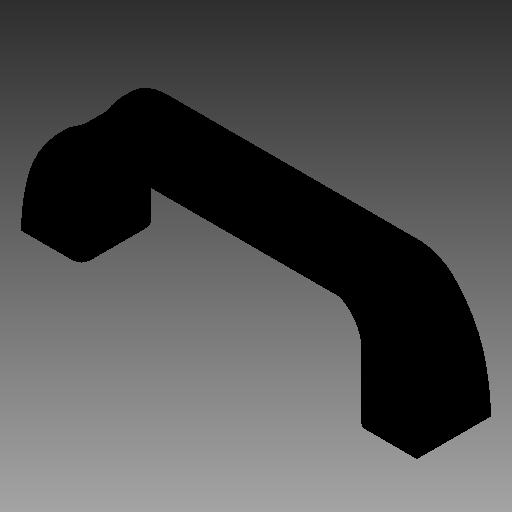
# Autodesk Inventor part: 2061
Saved by Autodesk Inventor 2019 (Build 230136000, 136)
## iProperties
Category: PARTsolutions
Company: 8020
Created: 2019-03-04
Part Number: 2061
Material: Generic
Catalog Web Link: www.cadenas.de
Description: 2060, 2061, 2062, 2880, 2881, 2882-Plastic Door Handles
Vendor: 8020
Document SubType Name: Modeling
Designer: psadmin
Manufacturer: 8020
Mass: 38.2907 g
Surface Area: 160.706 cm^2
Volume: 38.2907 cm^3
Density: 1 g/cm^3
Appearance: PSOLRGB-0-0-0
PSOL_IDENT_0: {$CADENAS_DATA\23d-libs\8020\inch\panels_and_doors\2060.prj},182 {VTYP=3D},{NB=2061},{LINA=2061},{NN=
PSOL_IDENT_1: 2060, 2061, 2062, 2880, 2881, 2882},{DATE=04.12.2018 10:30:17},{GEOMDATE=03.01.2012 00:00:00},{VERSI
PSOL_IDENT_2: ON=},{LINEID=300},{WBVAR=COLOR},{WBNUMERIC=}  {NB=2061},{LINA=2061},{KT=DUMMY},{PN=2061},{SIZE=Mediu
PSOL_IDENT_3: m},{MAT=High Strength Polycarbonate},{COLOR=Black},{A=5.473},{B=3.800},{C=1.614},{D=1.024},{E=4.607}
PSOL_IDENT_4: ,{F=5/16-18 SHCS (2)},{W=.095},{CC=8-15, 8-40},{COL=0.00,0.00,0.00,0.00}
NN: 2060, 2061, 2062, 2880, 2881, 2882
NT: Plastic Door Handles
NB: 2061
NBSYN: $PN.
LINA: 2061
PN: 2061
SIZE: Medium
MAT: High Strength Polycarbonate
COLOR: Black
A: 5.473
B: 3.8
C: 1.614
D: 1.024
E: 4.607
F: 5/16-18 SHCS (2)
W: .095
CC: 8-15, 8-40
SUPPLIER: 8020
ARTICLENO: 2061
BOMINFO: 2061
CREATOR: CADENAS GmbH
Title: 2061
Author: Cadenas PARTsolutions
Comments: Plastic Door Handles
Autodesk Inventor part; units mm, degrees
ref_plane "YZ Plane" through (0, 0, 0) normal (1, 0, 0) x (0, 1, 0)
ref_plane "XZ Plane" through (0, 0, 0) normal (0, 1, 0) x (-1, 0, 0)
ref_plane "XY Plane" through (0, 0, 0) normal (0, 0, 1) x (1, 0, 0)
sketch "Sketch_10" plane through (0, 0, 0) normal (0, 1, 0) x (-1, 0, 0)
  line L0 (21.2471, -13.0048) -> (21.2471, 13.0048)
  line L1 (21.2471, 13.0048) -> (3.0004, 13.0048)
  arc A0 (3.0004, 13.0048) -> (0, 10.0044) centre (3.0004, 10.0044) ccw
  line L2 (0, 10.0044) -> (0, -10.0044)
  arc A1 (0, -10.0044) -> (3.0004, -13.0048) centre (3.0004, -10.0044) ccw
  line L3 (3.0004, -13.0048) -> (21.2471, -13.0048)
  constraints: 8 end point, 4 point on circle, 2 centre point
extrude "Extrusion1" add sketch "Sketch_10" along normal blind 40.9956
sketch "Sketch_11" plane through (-21.2471, 0, 0) normal (1, 0, 0) x (0, 0, -1)
  arc A0 (-13.0048, 36.9951) -> (-10.0044, 33.9947) centre (-10.0044, 36.9951) ccw
  line L0 (-10.0044, 33.9947) -> (10.0044, 33.9947)
  arc A1 (10.0044, 33.9947) -> (13.0048, 36.9951) centre (10.0044, 36.9951) ccw
  line L1 (13.0048, 36.9951) -> (13.0048, 55.2418)
  line L2 (13.0048, 55.2418) -> (-13.0048, 55.2418)
  line L3 (-13.0048, 55.2418) -> (-13.0048, 36.9951)
  constraints: 8 end point, 4 point on circle, 2 centre point
extrude "Extrusion2" add sketch "Sketch_11" along normal blind 139.0142
sketch "Sketch_12" plane through (0, 0, 0) normal (0, 1, 0) x (-1, 0, 0)
  arc A0 (-96.52, 10.0044) -> (-99.5204, 13.0048) centre (-99.5204, 10.0044) ccw
  line L0 (-99.5204, 13.0048) -> (-117.7671, 13.0048)
  line L1 (-117.7671, 13.0048) -> (-117.7671, -13.0048)
  line L2 (-117.7671, -13.0048) -> (-99.5204, -13.0048)
  arc A1 (-99.5204, -13.0048) -> (-96.52, -10.0044) centre (-99.5204, -10.0044) ccw
  line L3 (-96.52, -10.0044) -> (-96.52, 10.0044)
  constraints: 8 end point, 4 point on circle, 2 centre point
extrude "Extrusion3" add sketch "Sketch_12" along normal blind 40.9956
sketch "Sketch_13" plane through (0, 23.0124, 0) normal (0, 1, 0) x (1, 0, 0)
  line L0 (12.1412, 10.0044) -> (12.1412, -10.0044)
  line L1 (-21.2471, 13.0048) -> (-21.2471, -13.0048)
  line L2 (-21.2471, -13.0048) -> (-3.0004, -13.0048)
  arc A0 (-3.0004, -13.0048) -> (0, -10.0044) centre (-3.0004, -10.0044) ccw
  line L3 (0, -10.0044) -> (0, 10.0044)
  arc A1 (0, 10.0044) -> (-3.0004, 13.0048) centre (-3.0004, 10.0044) ccw
  line L4 (-3.0004, 13.0048) -> (-21.2471, 13.0048)
  constraints: 10 end point, 4 point on circle, 2 centre point
revolve "Revolution1" add sketch "Sketch_13" angle 90 about axis through (12.1412, 23.0124, -10.0044) along (0, 0, -1)
sketch "Sketch_14" plane through (0, 23.0124, 0) normal (0, 1, 0) x (1, 0, 0)
  line L0 (84.3788, -10.0044) -> (84.3788, 10.0044)
  arc A0 (96.52, -10.0044) -> (99.5204, -13.0048) centre (99.5204, -10.0044) ccw
  line L1 (99.5204, -13.0048) -> (117.7671, -13.0048)
  line L2 (117.7671, -13.0048) -> (117.7671, 13.0048)
  line L3 (117.7671, 13.0048) -> (99.5204, 13.0048)
  arc A1 (99.5204, 13.0048) -> (96.52, 10.0044) centre (99.5204, 10.0044) ccw
  line L4 (96.52, 10.0044) -> (96.52, -10.0044)
  constraints: 10 end point, 4 point on circle, 2 centre point
revolve "Revolution2" add sketch "Sketch_14" angle 90 about axis through (84.3788, 23.0124, 10.0044) along (0, 0, 1)
sketch "Sketch_15" plane through (0, 0, 0) normal (0, 0, 1) x (1, 0, 0)
  line L0 (-33.9471, 81.9912) -> (-33.9471, 0)
  line L1 (-33.9471, 0) -> (-21.2471, 0)
  arc A0 (-19.4945, 15.0114) -> (-21.2471, 0) centre (51.2063, -0.851) ccw
  arc A1 (-9.9187, 34.0868) -> (-19.4945, 15.0114) centre (20.6584, 6.796) ccw
  arc A2 (3.0099, 40.9956) -> (-9.9187, 34.0868) centre (4.3058, 23.0194) ccw
  line L2 (3.0099, 40.9956) -> (93.5101, 40.9956)
  arc A3 (106.4387, 34.0868) -> (93.5101, 40.9956) centre (92.2142, 23.0194) ccw
  arc A4 (116.0145, 15.0114) -> (106.4387, 34.0868) centre (75.8616, 6.796) ccw
  arc A5 (117.7671, 0) -> (116.0145, 15.0114) centre (45.3137, -0.851) ccw
  line L3 (117.7671, 0) -> (130.4671, 0)
  line L4 (130.4671, 0) -> (130.4671, 81.9912)
  line L5 (130.4671, 81.9912) -> (-33.9471, 81.9912)
  constraints: 12 end point, 12 point on circle, 6 centre point
extrude "Extrusion4" cut sketch "Sketch_15" along normal mid plane 52.0192
sketch "Sketch_16" plane through (0, 0, 0) normal (0, 0, 1) x (1, 0, 0)
  line L0 (106.7689, 0) -> (106.7689, 40.9956)
  line L1 (106.7689, 40.9956) -> (113.2697, 40.9956)
  line L2 (113.2697, 40.9956) -> (113.2697, 6.0008)
  line L3 (113.2697, 6.0008) -> (111.0194, 6.0008)
  line L4 (111.0194, 6.0008) -> (111.0194, 0)
  line L5 (111.0194, 0) -> (106.7689, 0)
  line L6 (106.7689, 0) -> (106.7689, 40.9956)
  constraints: 14 end point
revolve "Revolution3" cut sketch "Sketch_16" angle 360 about axis through (106.7689, 0, 0) along (0, -1, 0)
sketch "Sketch_17" plane through (0, 0, 0) normal (0, 0, 1) x (1, 0, 0)
  line L0 (-10.2489, 0) -> (-10.2489, 40.9956)
  line L1 (-10.2489, 40.9956) -> (-3.7481, 40.9956)
  line L2 (-3.7481, 40.9956) -> (-3.7481, 6.0008)
  line L3 (-3.7481, 6.0008) -> (-5.9984, 6.0008)
  line L4 (-5.9984, 6.0008) -> (-5.9984, 0)
  line L5 (-5.9984, 0) -> (-10.2489, 0)
  line L6 (-10.2489, 0) -> (-10.2489, 40.9956)
  constraints: 14 end point
revolve "Revolution4" cut sketch "Sketch_17" angle 360 about axis through (-10.2489, 0, 0) along (0, -1, 0)
sketch "Sketch_18" plane through (0, 40.9956, 0) normal (0, 1, 0) x (1, 0, 0)
  line L0 (-33.9471, 25.7048) -> (-33.9471, -10.0013)
  line L1 (-33.9471, -10.0013) -> (-5.0206, -10.0013)
  arc A0 (-5.0206, -10.0013) -> (-3.0204, -8.001) centre (-5.0206, -8.001) ccw
  line L2 (-3.0204, -8.001) -> (-3.0204, 8.001)
  arc A1 (-3.0204, 8.001) -> (-5.0206, 10.0013) centre (-5.0206, 8.001) ccw
  line L3 (-5.0206, 10.0013) -> (-21.2471, 10.0013)
  line L4 (-21.2471, 10.0013) -> (-21.2471, 13.0048)
  line L5 (-21.2471, 13.0048) -> (117.7671, 13.0048)
  line L6 (117.7671, 13.0048) -> (117.7671, 10.0013)
  line L7 (117.7671, 10.0013) -> (101.5406, 10.0013)
  arc A2 (101.5406, 10.0013) -> (99.5404, 8.001) centre (101.5406, 8.001) ccw
  line L8 (99.5404, 8.001) -> (99.5404, -8.001)
  arc A3 (99.5404, -8.001) -> (101.5406, -10.0013) centre (101.5406, -8.001) ccw
  line L9 (101.5406, -10.0013) -> (130.4671, -10.0013)
  line L10 (130.4671, -10.0013) -> (130.4671, 25.7048)
  line L11 (130.4671, 25.7048) -> (-33.9471, 25.7048)
  constraints: 24 end point, 8 point on circle, 4 centre point
extrude "Extrusion5" cut sketch "Sketch_18" against normal blind 26.0032
body "Solid1"
